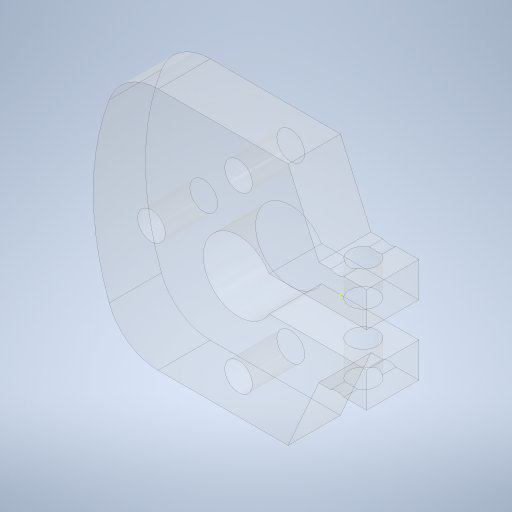
# Autodesk Inventor part: 射出_腕固定2_真
Saved by Autodesk Inventor 2023 (Build 270158000, 158)
## iProperties
Created: 2022-04-21
Part Number: 射出_腕固定2_真
Material: ポリカーボネート、クリア
Document SubType Name: Modeling
Designer: yuta
Density: 1.2 g/cm^3
Appearance: ポリカーボネート - クリア
Author: yuta
Autodesk Inventor part; units mm, degrees
ref_plane "YZ Plane" through (0, 0, 0) normal (1, 0, 0) x (0, 1, 0)
ref_plane "XZ Plane" through (0, 0, 0) normal (0, 1, 0) x (-1, 0, 0)
ref_plane "XY Plane" through (0, 0, 0) normal (0, 0, 1) x (1, 0, 0)
sketch "スケッチ1" plane through (0, 0, 0) normal (0, 0, 1) x (1, 0, 0)
  line L0 (9, 0) -> (9, 4)
  line L1 (9, 12) -> (2.2731, 12)
  line L2 (0, 8) -> (9, 8)
  line L3 (0, 4) -> (9, 4)
  line L4 (9, 8) -> (9, 12)
  line L5 (2.2731, 12) -> (0, 14.2779)
  line L6 (2.2731, 0) -> (-5.7099, -8)
  line L7 (-5.7099, 20) -> (-15.7099, 20)
  line L8 (-5.7099, -8) -> (-15.7099, -8)
  line L9 (-15.7099, 20) -> (-25.7698, 20)
  line L10 (-25.7698, 20) -> (-25.7698, -8)
  line L11 (-25.7698, -8) -> (-15.7099, -8)
  line L12 (2.2731, 0) -> (9, 0)
  line L13 (0, 14.2779) -> (-5.7099, 20)
  arc A0 (-2.1881, 8) -> (-2.1881, 4) centre (-5.7099, 6) ccw
  line L14 (0, 8) -> (-2.1881, 8)
  line L15 (0, 4) -> (-2.1881, 4)
  point P0 (0, 0)
  point P1 (4.5, 12)
  point P2 (4.5, 0)
  point P3 (4.5, 4)
  point P4 (-25.7099, 6)
  dimension "d5" = 4
  dimension "d8" = 10
  dimension "d9" = 10
  dimension "d12" = 14
  dimension "d90" = 8.1
  constraints: 32 end point, 6 horizontal, 6 perpendicular, 2 parallel, 2 point on circle, 1 centre point, 1 midpoint, 1 point on line
  measures "d5" distance between parallel lines of L3 L2
  measures "d8" distance of L7.start L7.end
  measures "d9" distance of L6.end L8.end
  measures "d12" distance from line of L8 point (-25.71, 6)
  measures "d90" diameter of A0
extrude "押し出し1" add sketch "スケッチ1" along normal blind 6
sketch "スケッチ2" plane through (0, 0, 6) normal (0, 0, 1) x (1, 0, 0)
  circle A0 centre (5.6365, 13.3) radius 1.5
  line L0 (9, 8) -> (9, 12) projected
  line L1 (11.5477, 6) -> (-28.1936, 6) construction
  line L2 (9, 12) -> (2.2731, 12) projected
  circle A1 centre (5.6365, -1.3) radius 1.5
  point P0 (0, 0)
  point P1 (4.8882, 12)
  point P2 (6.3849, 12)
  dimension "d15" = 3
  dimension "d16" = 3.3635
  dimension "d17" = 1.3
  constraints: 2 centre point, 2 end point, 1 horizontal, 1 symmetric about line, 1 other
  measures "d15" diameter of A0
  measures "d16" distance from line of L0 A0.centre
  measures "d17" distance from line of L2 A0.centre
extrude "押し出し2" cut sketch "スケッチ2" against normal blind 6 contours A0 L2 | A1 picked at (5.4614, 13.0013)
sketch "スケッチ3" plane through (0, 0, 6) normal (0, 0, 1) x (1, 0, 0)
  circle A0 centre (5.6365, 13.3) radius 1.5
  line L0 (9, 12) -> (2.2731, 12) projected
  point P0 (0, 0)
  point P1 (4.8882, 12)
  point P2 (6.3849, 12)
  dimension "d20" = 3
  dimension "d21" = 1.3
  constraints: 1 centre point
  measures "d20" diameter of A0
  measures "d21" distance from line of L0 A0.centre
extrude "押し出し3" add sketch "スケッチ3" against normal blind 6 contours A0 L0 picked at (5.4614, 13.0013)
sketch "スケッチ4" plane through (0, 0, 6) normal (0, 0, 1) x (1, 0, 0)
  arc A0 (6.3849, 12) -> (4.8882, 12) centre (5.6365, 13.3) ccw projected
  circle A1 centre (5.6365, 13.3) radius 1.5
  point P0 (0, 0)
  dimension "d24" = 3
  constraints: 1 centre point, 1 coincident
  measures "d24" diameter of A1
extrude "押し出し4" cut sketch "スケッチ4" against normal blind 6
fillet "フィレット1" radius 5 1 edges at (-25.7698, 20, 3)
fillet "フィレット2" radius 5 1 edges at (-25.7698, -8, 3)
fillet "フィレット3" radius 3 4 edges at (-5.7099, -8, 3) (2.2731, 0, 3) (-5.7099, 20, 3) (2.2731, 12, 3)
sketch "スケッチ6" plane through (0, 4, 0) normal (0, 1, 0) x (1, 0, 0)
  point P0 (0, 0)
sketch "スケッチ7" plane through (4.8882, 12, 6) normal (0, 1, 0) x (1, 0, 0)
  circle A0 centre (0.7488, 3) radius 1.6
  line L0 (1.4967, 0) -> (0, 0) projected
  line L1 (4.1118, 6) -> (4.1118, 0) projected
  point P0 (-4.8882, 6)
  point P1 (0.7483, 0)
  dimension "d43" = 3.2
  dimension "d44" = 3
  dimension "d45" = 3.363
  constraints: 1 centre point, 1 midpoint
  measures "d43" diameter of A0
  measures "d44" distance of A0.centre point (0.748, 0)
  measures "d45" distance from line of L1 A0.centre
extrude "押し出し5" cut sketch "スケッチ7" against normal blind 28
sketch "スケッチ11" plane through (0, 0, 6) normal (0, 0, 1) x (1, 0, 0)
  line L0 (-6.9544, 20) -> (-20.7698, 20) projected
  line L1 (-20.7698, 20) -> (-6.9544, 20)
  arc A0 (1.394, 12.8809) -> (3.5176, 12) centre (3.5176, 15) ccw projected
  line L2 (0, 20) -> (1.3068, 17.0279)
  arc A1 (1.394, 12.8809) -> (3.5176, 12) centre (3.5176, 15) ccw
  arc A2 (-4.8308, 19.1191) -> (-6.9544, 20) centre (-6.9544, 17) ccw projected
  arc A3 (-4.8308, 19.1191) -> (-6.9544, 20) centre (-6.9544, 17) ccw
  line L3 (1.394, 12.8809) -> (-4.8308, 19.1191) projected
  line L4 (-4.8308, 19.1191) -> (1.394, 12.8809)
  arc A4 (0, 8) -> (0, 4) centre (-5.7099, 6) ccw projected
  line L5 (-11.7599, 6) -> (12.1155, 6) construction
  line L6 (-20.7698, -8) -> (0, -8)
  line L7 (0, -8) -> (3.5176, 0)
  arc A5 (-6.9544, -8) -> (-4.8308, -7.1191) centre (-6.9544, -5) ccw
  line L8 (1.394, -0.8809) -> (-4.8308, -7.1191)
  line L9 (-6.9544, 20) -> (0, 20)
  line L10 (1.3068, 17.0279) -> (3.5176, 12)
  arc A6 (3.5176, 0) -> (1.394, -0.8809) centre (3.5176, -3) ccw
  point P0 (0, 0)
  constraints: 19 end point, 9 point on circle, 7 symmetric about line, 4 centre point, 3 horizontal, 2 coincident, 2 tangent, 1 collinear, 1 concentric, 1 point on line, 1 other
extrude "押し出し6" add sketch "スケッチ11" against normal blind 6
sketch "スケッチ12" plane through (0, 0, 6) normal (0, 0, 1) x (1, 0, 0)
  arc A0 (0, 8) -> (0, 4) centre (-5.7099, 6) ccw projected
  point P0 (0, 0)
  point P1 (-15.7099, 6)
  point P2 (-5.7099, 16)
  point P3 (-5.7099, -4)
  dimension "d74" = 10
  dimension "d76" = 10
  dimension "d77" = 10
  measures "d74" distance of point (-15.71, 6) A0.centre
  measures "d76" distance of A0.centre point (-5.71, 16)
  measures "d77" distance of point (-5.71, -4) A0.centre
hole "穴4" at (-15.7099, 6, 6) at (-5.7099, 16, 6) at (-5.7099, -4, 6) direction (0, 0, -1) diameter 3.2 end through all
sketch "スケッチ13" plane through (0, 0, 6) normal (0, 0, 1) x (1, 0, 0)
  line L0 (-20.7698, -8) -> (0, -8) projected
  line L1 (0, 20) -> (-20.7698, 20) projected
  line L2 (-18.7698, 20) -> (-18.7698, -8) construction
  line L3 (-25.7698, 15) -> (-25.7698, -3) projected
  arc A0 (-18.7698, 20) -> (-18.7698, -8) centre (6.3784, 6) ccw
  line L4 (-18.7698, 20) -> (-29.3351, 20)
  line L5 (-29.3351, 20) -> (-29.3351, -8)
  line L6 (-29.3351, -8) -> (-18.7698, -8)
  point P0 (0, 0)
  dimension "d85" = 7
  constraints: 8 end point, 2 perpendicular, 2 point on circle, 2 point on line, 1 centre point, 1 horizontal
  measures "d85" distance between parallel lines of L3 L2
extrude "押し出し7" cut sketch "スケッチ13" against normal blind 6
fillet "フィレット4" radius 6 1 edges at (-18.7698, 20, 3)
fillet "フィレット5" radius 6 1 edges at (-18.7698, -8, 3)
